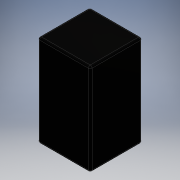
# Autodesk Inventor part: Toggle_Base
Saved by Autodesk Inventor 2016 (Build 200138000, 138)
## iProperties
Created: 2016-04-13
Part Number: Toggle_Base
Material: PC/ABS Plastic
Document SubType Name: Modeling
Designer: agmle
Density: 0.357273 g/cm^3
Appearance: Smooth - Black
Author: agmle
Autodesk Inventor part; units mm, degrees
ref_plane "YZ Plane" through (0, 0, 0) normal (1, 0, 0) x (0, 1, 0)
ref_plane "XZ Plane" through (0, 0, 0) normal (0, 1, 0) x (-1, 0, 0)
ref_plane "XY Plane" through (0, 0, 0) normal (0, 0, 1) x (1, 0, 0)
sketch "Sketch1" plane through (0, 0, 0) normal (0, 1, 0) x (-1, 0, 0)
  line L0 (7, 12.25) -> (-7, 12.25)
  line L1 (-7, 12.25) -> (-7, -12.25)
  line L2 (-7, -12.25) -> (7, -12.25)
  line L3 (7, -12.25) -> (7, 12.25)
  line L4 (7, 0) -> (-7, 0) construction
  point P0 (0, 0)
  point P1 (0, 0)
  dimension "d0" = 14
  dimension "d1" = 24.5
  constraints: 10 end point, 3 midpoint, 2 parallel, 1 coincident, 1 horizontal, 1 perpendicular
  measures "d0" distance of L0.start L0.end
  measures "d1" distance of L2.end L0.start
extrude "Extrusion1" add sketch "Sketch1" along normal blind 13.88
fillet "Fillet1" radius 0.5 12 edges at (7, 6.94, 12.25) (-7, 6.94, 12.25) (-7, 6.94, -12.25) (7, 6.94, -12.25) (7, 13.88, 0) (0, 13.88, -12.25) (-7, 13.88, 0) (0, 13.88, 12.25) (0, 0, 12.25) (7, 0, 0) (0, 0, -12.25) (-7, 0, 0)
body "Solid1"
